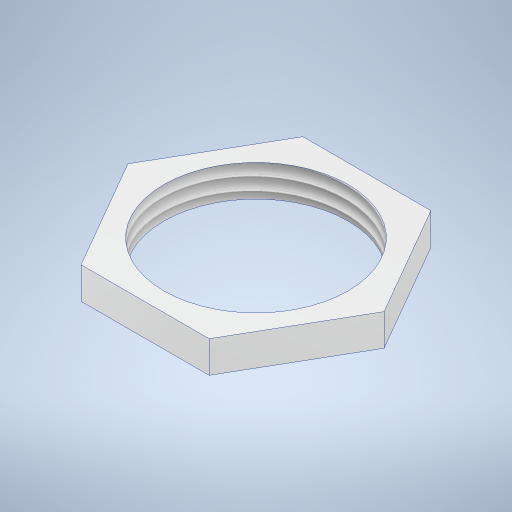
# Autodesk Inventor part: KeyLockNut
Saved by Autodesk Inventor 2024 (Build 280153000, 153)
## iProperties
Created: 2023-06-10
Part Number: KeyLockNut
Material: Generic
Document SubType Name: Modeling
Designer: 18179
Density: 1 g/cm^3
Appearance: Aluminum - Flat
Author: 18179
Autodesk Inventor part; units mm, degrees
ref_plane "YZ Plane" through (0, 0, 0) normal (1, 0, 0) x (0, 1, 0)
ref_plane "XZ Plane" through (0, 0, 0) normal (0, 1, 0) x (-1, 0, 0)
ref_plane "XY Plane" through (0, 0, 0) normal (0, 0, 1) x (1, 0, 0)
sketch "Sketch1" plane through (0, 0, 0) normal (0, 1, 0) x (-1, 0, 0)
  line L0 (6.4158, 11.1125) -> (12.8316, 0)
  line L1 (12.8316, 0) -> (6.4158, -11.1125)
  line L2 (6.4158, -11.1125) -> (-6.4158, -11.1125)
  line L3 (-6.4158, -11.1125) -> (-12.8316, 0)
  line L4 (-12.8316, 0) -> (-6.4158, 11.1125)
  line L5 (-6.4158, 11.1125) -> (6.4158, 11.1125)
  circle A0 centre (0, 0) radius 9.2329
  point P0 (0, 11.1125)
  dimension "d0" = 11.1125
  dimension "d1" = 18.4658
  constraints: 12 end point, 2 coincident, 1 centre point, 1 midpoint, 13 other
  measures "d0" distance of point (0, 11.113) point (0, 0)
  measures "d1" diameter of A0
extrude "Extrusion1" add sketch "Sketch1" along normal blind 3.175
thread "Thread1" size "3/4-20 UNEF" class "2B" standard "ANSI Unified Screw Threads" full length
body "Solid1"
